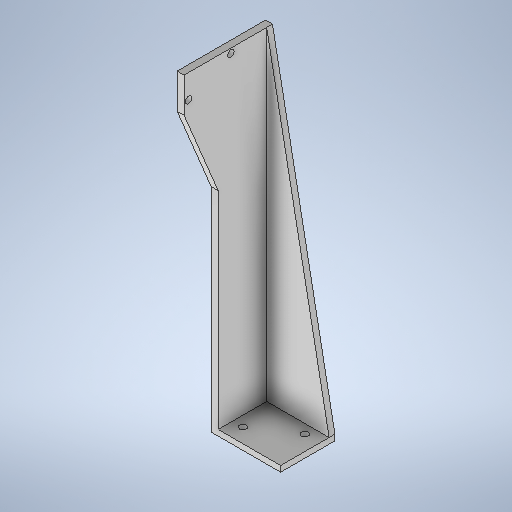
# Autodesk Inventor part: LimitSwitchBottomV3
Saved by Autodesk Inventor 2025.1 (Build 291241020, 241B)
## iProperties
Created: 2025-04-13
Part Number: LimitSwitchBottomV3
Material: Generic
Document SubType Name: Modeling
Designer: dpseu
Density: 1 g/cm^3
Appearance: Default
Author: dpseu
Autodesk Inventor part; units mm, degrees
ref_plane "YZ Plane" through (0, 0, 0) normal (1, 0, 0) x (0, 1, 0)
ref_plane "XZ Plane" through (0, 0, 0) normal (0, 1, 0) x (-1, 0, 0)
ref_plane "XY Plane" through (0, 0, 0) normal (0, 0, 1) x (1, 0, 0)
sketch "Sketch1" plane through (0, 0, 0) normal (0, 1, 0) x (-1, 0, 0)
  line L0 (0, 0) -> (29.7942, 0)
  line L1 (29.7942, 0) -> (29.7942, -38.1)
  line L2 (29.7942, -38.1) -> (0, -38.1)
  line L3 (0, -38.1) -> (0, 0)
  circle A0 centre (21.844, -9.525) radius 1.905
  circle A1 centre (8.255, -29.845) radius 1.905
  dimension "d0" = 29.7942
  dimension "d1" = 38.1
  dimension "d2" = 3.81
  dimension "d3" = 3.81
  dimension "d4" = 7.9502
  dimension "d5" = 9.525
  dimension "d6" = 8.255
  dimension "d7" = 8.255
  constraints: 8 end point, 2 centre point, 2 parallel, 1 horizontal, 1 perpendicular
  measures "d0" distance of L1.end L2.end
  measures "d1" distance of L0.end L1.end
  measures "d2" diameter of A0
  measures "d3" diameter of A1
  measures "d4" distance from line of L1 A0.centre
  measures "d5" distance from line of L0 A0.centre
  measures "d6" distance from line of L2 A1.centre
  measures "d7" distance from line of L3 A1.centre
extrude "Extrusion1" add sketch "Sketch1" along normal blind 3.175
sketch "Sketch2" plane through (-29.7942, 0, 0) normal (0, 0, 1) x (1, 0, 0)
  line L0 (29.7942, 0) -> (0, 0) projected
  line L1 (0, 0) -> (29.7942, 0)
  line L2 (29.7942, 0) -> (29.7942, -177.8)
  line L3 (29.7942, -177.8) -> (0, -177.8)
  line L4 (0, -113.5257) -> (0, 0)
  circle A0 centre (6.9723, -175.3108) radius 1.8034
  circle A1 centre (-16.2433, -164.7952) radius 1.8034
  line L5 (0, -177.8) -> (-18.7325, -177.8)
  line L6 (-18.7325, -177.8) -> (-18.7325, -158.75)
  line L7 (-18.7325, -158.75) -> (0, -113.5257)
  dimension "d11" = 177.8
  dimension "d12" = 3.6068
  dimension "d13" = 3.6068
  dimension "d15" = 13.0048
  dimension "d16" = 2.4892
  dimension "d22" = 157.5
  dimension "d24" = 19.05
  dimension "d25" = 48.5267
  dimension "d26" = 29.7942
  dimension "d27" = 2.4892
  dimension "d28" = 25.7048
  constraints: 14 end point, 2 centre point, 2 horizontal, 2 parallel, 2 perpendicular
  measures "d11" distance of L1.end L2.end
  measures "d12" diameter of A0
  measures "d13" diameter of A1
  measures "d15" distance from line of L3 A1.centre
  measures "d16" distance from line of L3 A0.centre
  measures "d22" angle of L7 L6
  measures "d24" distance of L5.end L6.end
  measures "d25" distance between parallel lines of L6 L2
  measures "d26" distance between parallel lines of L4 L2
  measures "d27" distance from line of L6 A1.centre
  measures "d28" distance from line of L6 A0.centre
extrude "Extrusion2" add sketch "Sketch2" against normal blind 3.81
sketch "Sketch3" plane through (0, 3.175, 0) normal (1, 0, 0) x (0, 0, -1)
  line L0 (3.81, -3.175) -> (3.81, -180.975) projected
  line L1 (38.1, -3.175) -> (3.81, -180.975)
  line L2 (38.1, -3.175) -> (3.81, -3.175)
  point P0 (0, -3.175)
  constraints: 4 end point, 1 horizontal
extrude "Extrusion3" add sketch "Sketch3" against normal blind 3.175
body "Solid1"
